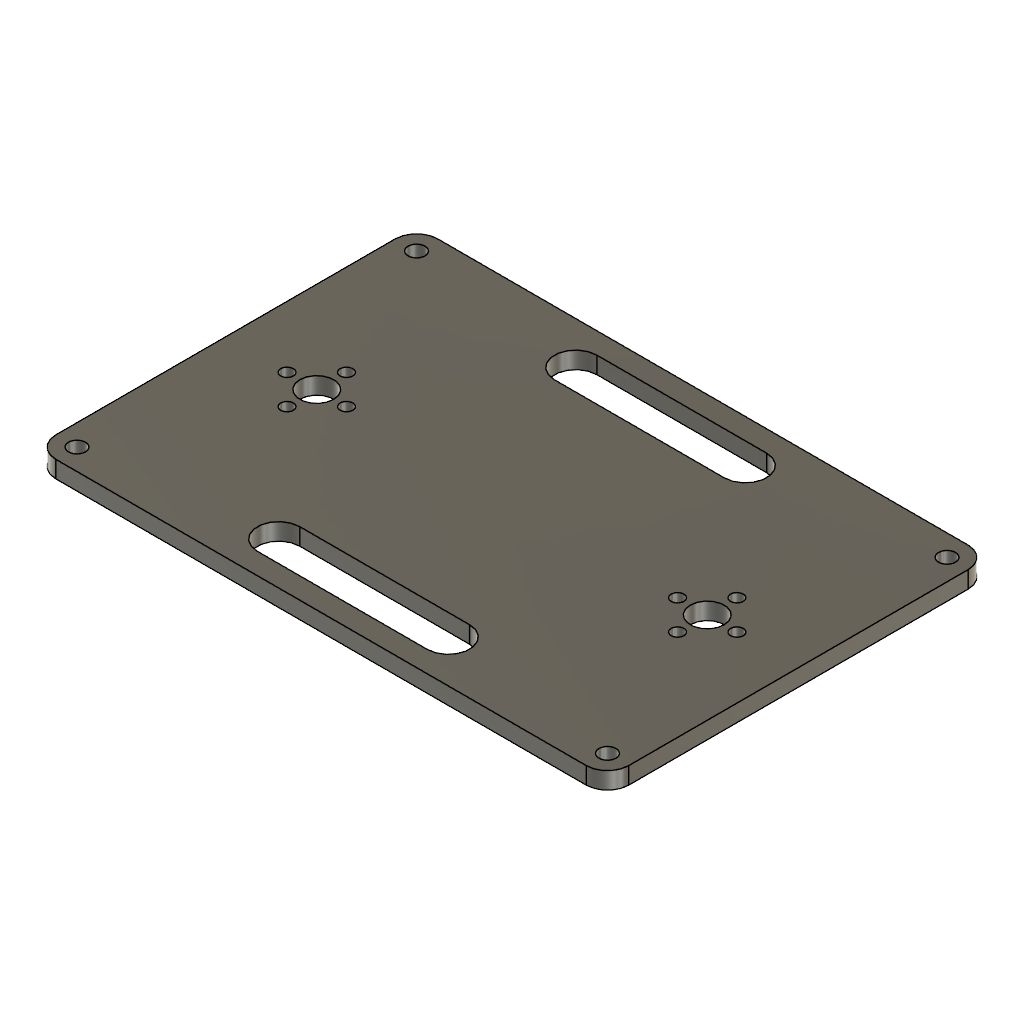
BASE_BALANCIN (Autodesk Fusion 360 design; units mm, degrees)
Autodesk Fusion 360 part; units mm, degrees
note: some values were not read from the file. Set by a fixed rule: which sketch regions a step uses.
sketch "Boceto1" plane through (0, 0, 0) normal (0, 0, 1) x (1, 0, 0)
  line L0 (-67.5, 45) -> (67.5, 45)
  line L1 (67.5, 45) -> (67.5, -45)
  line L2 (67.5, -45) -> (-67.5, -45)
  line L3 (-67.5, -45) -> (-67.5, 45)
  line L4 (-67.5, 45) -> (67.5, -45) construction
  line L5 (67.5, 45) -> (-67.5, -45) construction
  dimension "d1" = 135
  dimension "d2" = 90
  constraint horizontal L0
  constraint perpendicular L0 L1
  constraint parallel L0 L2
  constraint parallel L1 L3
  constraint coincident L4 origin
  constraint coincident L5 origin
  measures "d1" distance of L1.end L2.end
extrude "Extruir1" add sketch "Boceto1" along normal blind 4
sketch "Boceto2" plane through (0, 0, 4) normal (0, 0, 1) x (-1, 0, 0)
  line L0 (67.5, 45) -> (-67.5, 45)
  line L1 (-67.5, 45) -> (-67.5, -45)
  line L2 (-67.5, -45) -> (67.5, -45)
  line L3 (67.5, -45) -> (67.5, 45)
  line L4 (67.5, -45) -> (67.5, -40)
  line L5 (67.5, -40) -> (62.5, -40)
  line L6 (67.5, 45) -> (62.5, 45)
  line L7 (62.5, 45) -> (62.5, 40)
  line L8 (-67.5, -45) -> (-62.5, -45)
  line L9 (-62.5, -45) -> (-62.5, -40)
  line L10 (-67.5, 45) -> (-67.5, 40)
  line L11 (-67.5, 40) -> (-62.5, 40)
  circle A0 centre (62.5, -40) radius 2
  circle A1 centre (62.5, 40) radius 2
  circle A2 centre (-62.5, -40) radius 2
  circle A3 centre (-62.5, 40) radius 2
  dimension "d5" = 5
  dimension "d6" = 5
  dimension "d7" = 135
  dimension "d8" = 90
  dimension "d9" = 5
  dimension "d10" = 5
  dimension "d11" = 5
  dimension "d12" = 5
  dimension "d13" = 5
  dimension "d14" = 5
  dimension "d15" = 4
  dimension "d16" = 4
  dimension "d17" = 4
  dimension "d18" = 4
  constraint coincident L2.end L3.start
  constraint perpendicular L2 L4
  constraint perpendicular L3 L5
  constraint coincident L0.start L3.end
  constraint perpendicular L3 L6
  constraint perpendicular L0 L7
  constraint coincident L1.end L2.start
  constraint perpendicular L1 L8
  constraint perpendicular L2 L9
  constraint coincident L0.end L1.start
  constraint perpendicular L0 L10
  constraint perpendicular L1 L11
  constraint coincident L5.end A0.centre
  constraint coincident L7.end A1.centre
  constraint coincident L9.end A2.centre
  constraint coincident L11.end A3.centre
  measures "d1" distance of L1.end L2.end
extrude "Extruir2" cut sketch "Boceto2" against normal blind 4 contours A0 | A1 | A2 | A3
fillet "Empalme1" radius 5 4 edges at (-67.5, -45, 2) (67.5, -45, 2) (67.5, 45, 2) (-67.5, 45, 2)
sketch "Boceto3" plane through (0, 0, 4) normal (0, 0, 1) x (-1, 0, 0)
  circle A0 centre (62.5, 40) radius 2
  circle A1 centre (-62.5, -40) radius 2
  circle A2 centre (62.5, -40) radius 2
  circle A3 centre (-62.5, 40) radius 2
  arc A4 (62.5, -45) -> (67.5, -40) centre (62.5, -40) ccw
  line L0 (67.5, -40) -> (67.5, 40)
  arc A5 (67.5, 40) -> (62.5, 45) centre (62.5, 40) ccw
  line L1 (62.5, 45) -> (-62.5, 45)
  arc A6 (-62.5, 45) -> (-67.5, 40) centre (-62.5, 40) ccw
  line L2 (-67.5, 40) -> (-67.5, -40)
  arc A7 (-67.5, -40) -> (-62.5, -45) centre (-62.5, -40) ccw
  line L3 (-62.5, -45) -> (62.5, -45)
  line L4 (-67.5, 0) -> (-46, 0)
  circle A8 centre (-46, 0) radius 4
  circle A9 centre (-46, 0) radius 7
  line L5 (-46, 0) -> (-46, -7) construction
  line L6 (-46, 0) -> (-39, 0) construction
  line L7 (-46, 0) -> (-46, 7) construction
  line L8 (-46, 0) -> (-53, 0) construction
  circle A10 centre (-46, -7) radius 1.5
  circle A11 centre (-39, 0) radius 1.5
  circle A12 centre (-46, 7) radius 1.5
  circle A13 centre (-53, 0) radius 1.5
  dimension "d23" = 21.5
  dimension "d24" = 8
  dimension "d25" = 14
  dimension "d26" = 3
  dimension "d27" = 3
  dimension "d28" = 3
  dimension "d29" = 3
  constraint midpoint L2 L4.start
  constraint perpendicular L2 L4
  constraint coincident L4.end A8.centre
  constraint concentric A8 A9
  constraint coincident A9 L5.end
  constraint perpendicular L4 L5
  constraint coincident A9 L6.end
  constraint perpendicular L5 L6
  constraint coincident A9 L7.end
  constraint perpendicular L6 L7
  constraint coincident L4 L8.end
  constraint coincident A9 L8.end
  constraint coincident L5.end A10.centre
  constraint coincident L6.end A11.centre
  constraint coincident L7.end A12.centre
  constraint coincident L8.end A13.centre
  measures "d23" distance of L4.start L4.end
  measures "d24" diameter of A8
  measures "d25" diameter of A9
  measures "d26" diameter of A10
  measures "d27" diameter of A11
  measures "d28" diameter of A12
  measures "d29" diameter of A13
extrude "Extruir3" cut sketch "Boceto3" against normal blind 4 contours L4 A9 A13 | L4 A9 A13 | L4 A9 A13 | L4 A9 A13 | A9 A12 | A9 A12 | A9 A10 | A9 A10 | A9 A11 | A9 A11 | A8
mirror "Simetría1" about plane through (0, 0, 0) normal (1, 0, 0) of "Extruir3"
sketch "Boceto4" plane through (0, 0, 4) normal (0, 0, 1) x (-1, 0, 0)
  circle A0 centre (46, 7) radius 1.5
  circle A1 centre (46, -7) radius 1.5
  circle A2 centre (39, 0) radius 1.5
  circle A3 centre (53, 0) radius 1.5
  circle A4 centre (46, 0) radius 4
  arc A5 (62.5, -45) -> (67.5, -40) centre (62.5, -40) ccw
  line L0 (67.5, -40) -> (67.5, 40)
  arc A6 (67.5, 40) -> (62.5, 45) centre (62.5, 40) ccw
  line L1 (62.5, 45) -> (-62.5, 45)
  arc A7 (-62.5, 45) -> (-67.5, 40) centre (-62.5, 40) ccw
  line L2 (-67.5, 40) -> (-67.5, -40)
  arc A8 (-67.5, -40) -> (-62.5, -45) centre (-62.5, -40) ccw
  line L3 (-62.5, -45) -> (62.5, -45)
  circle A9 centre (-62.5, 40) radius 2
  circle A10 centre (62.5, -40) radius 2
  circle A11 centre (-62.5, -40) radius 2
  circle A12 centre (62.5, 40) radius 2
  circle A13 centre (-46, 7) radius 1.5
  circle A14 centre (-46, -7) radius 1.5
  circle A15 centre (-53, 0) radius 1.5
  circle A16 centre (-39, 0) radius 1.5
  circle A17 centre (-46, 0) radius 4
  line L4 (0, 35) -> (0, -35)
  line L5 (-20, -35) -> (20, -35)
  line L6 (-20, 35) -> (20, 35)
  line L7 (20, -30) -> (-20, -30)
  arc A18 (-20, -30) -> (-20, -40) centre (-20, -35) ccw
  line L8 (-20, -40) -> (20, -40)
  arc A19 (20, -40) -> (20, -30) centre (20, -35) ccw
  line L9 (20, -35) -> (-20, -35) construction
  line L10 (20, 40) -> (-20, 40)
  arc A20 (-20, 40) -> (-20, 30) centre (-20, 35) ccw
  line L11 (-20, 30) -> (20, 30)
  arc A21 (20, 30) -> (20, 40) centre (20, 35) ccw
  line L12 (20, 35) -> (-20, 35) construction
  dimension "d34" = 70
  dimension "d35" = 40
  dimension "d36" = 40
  dimension "d37" = 10
  dimension "d38" = 10
  constraint midpoint L4 origin
  constraint vertical L4
  constraint midpoint L4.end L5
  constraint perpendicular L4 L5
  constraint midpoint L4.start L6
  constraint perpendicular L4 L6
  constraint tangent L7 A18
  constraint tangent A18 L8
  constraint parallel L7 L8
  constraint tangent L8 A19
  constraint tangent L7 A19
  constraint coincident L5.start A18.centre
  constraint perpendicular L4 L9
  constraint coincident L5.end A19.centre
  constraint tangent L10 A20
  constraint tangent A20 L11
  constraint parallel L10 L11
  constraint tangent L11 A21
  constraint tangent L10 A21
  constraint coincident L6.start A20.centre
  constraint perpendicular L4 L12
  constraint coincident L6.end A21.centre
  measures "d34" distance of L4.start L4.end
  measures "d35" distance of L5.start L5.end
  measures "d36" distance of L6.start L6.end
  measures "d37" diameter of A18
  measures "d38" diameter of A20
extrude "Extruir4" cut sketch "Boceto4" against normal blind 4 contours L7 A18 L8 A19 | L10 A20 L11 A21
